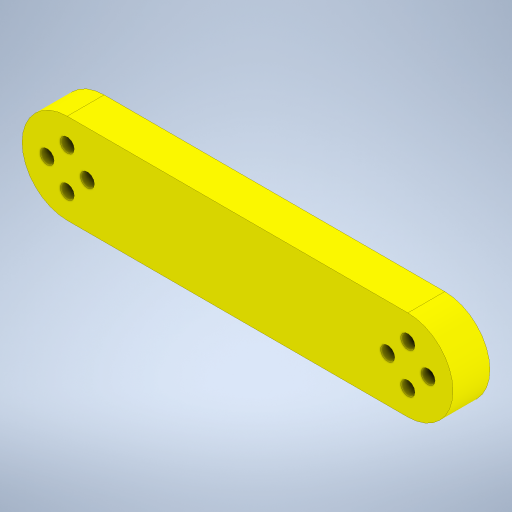
# Autodesk Inventor part: Ramie2
Saved by Autodesk Inventor 2024.2 (Build 282272000, 272)
## iProperties
Created: 2023-11-11
Part Number: Ramie2
Material: Ogólny
Document SubType Name: Modeling
Designer: nosal
Density: 1 g/cm^3
Appearance: Domyślna
Author: nosal
## iProperties of the stored document Ramie2_Drukowanie 3D.ipt
Created: 2023-11-12
Part Number: Ramie2_Drukowanie 3D
Material: Ogólny
Document SubType Name: Modeling
Designer: nosal
Density: 1 g/cm^3
Appearance: Domyślna
Author: nosal
Autodesk Inventor part; units mm, degrees
ref_plane "YZ Plane" through (0, 0, 0) normal (1, 0, 0) x (0, 1, 0)
ref_plane "XZ Plane" through (0, 0, 0) normal (0, 1, 0) x (-1, 0, 0)
sketch "Szkic1" plane through (0, 0, 0) normal (0, 0, 1) x (1, 0, 0)
  circle A0 centre (0, 0) radius 3.5
  circle A1 centre (0, 0) radius 15.9
  circle A2 centre (0, 0) radius 11.5
  line L0 (0, -15.9) -> (-60, -15.9)
  line L1 (0, 15.9) -> (-60, 15.9)
  line L2 (-60, 15.9) -> (-60, -15.9)
  point P0 (0, 7.1)
  point P1 (-7.1, 0)
  point P2 (7.1, 0)
  point P3 (0, -7.1)
  dimension "d0" = 7
  dimension "d1" = 7.1
  dimension "d2" = 7.1
  dimension "d3" = 7.1
  dimension "d4" = 7.1
  dimension "d5" = 31.8
  dimension "d6" = 23
  dimension "d23" = 60
  constraints: 6 end point, 3 centre point, 3 coincident, 2 horizontal, 2 point on circle, 1 perpendicular, 1 tangent
  measures "d0" diameter of A0
  measures "d1" distance of point (0, 0) point (0, 7.1)
  measures "d2" distance of point (7.1, 0) point (0, 0)
  measures "d3" distance of point (0, -7.1) point (0, 0)
  measures "d4" distance of point (-7.1, 0) point (0, 0)
  measures "d5" diameter of A1
  measures "d6" diameter of A2
  measures "d23" distance of L0.start L0.end
extrude "Wyciągnięcie proste1" add sketch "Szkic1" along normal blind 10 contours A0 | A1 | A1 L0 L2 L1 | A2
extrude "Wyciągnięcie proste2" cut sketch "Szkic1" along normal blind 2 contours A2
extrude "Wyciągnięcie proste3" cut sketch "Szkic1" along normal blind 3 contours A0
hole "Otwór1" at (0, 7.1, 0) at (-7.1, 0, 0) at (7.1, 0, 0) at (0, -7.1, 0) direction (0, 0, 1) diameter 1.567 end through all thread size "M2x0.4" designation "M2" class "6H" standard "GB Metric profile"
sketch "Szkic2" plane through (0, 0, 0) normal (0, 0, -1) x (0, -1, 0)
  arc A0 (-15.9, 0) -> (15.9, 0) centre (0, 0) ccw projected
  circle A1 centre (0, 0) radius 11.5 projected
  circle A2 centre (0, 0) radius 13.9
  line L0 (15.9, 60) -> (15.9, 0) projected
  line L1 (-15.9, 60) -> (15.9, 60) projected
  line L2 (-15.9, 0) -> (-15.9, 60) projected
  dimension "d20" = 2
  constraints: 1 centre point
  measures "d20" radial gap between concentric circles of A0 A2
extrude "Wyciągnięcie proste4" add sketch "Szkic2" along normal blind 3 contours L2 L1 L0 A0
ref_plane "Płaszczyzna konstrukcyjna2" through (-60, 15.9, 10) normal (1, 0, 0) x (0, -1, 0)
mirror "Odbij1" about plane through (-60, 15.9, 0) normal (-1, 0, 0) of "Wyciągnięcie proste4", "Otwór1", "Wyciągnięcie proste1", "Wyciągnięcie proste2"
sketch "Szkic4" plane through (-120, 0, 0) normal (0, 0, -1) x (-1, 0, 0)
  circle A0 centre (0, 0) radius 3.5 projected
  point P0 (-120, 0)
extrude "Wyciągnięcie proste5" cut sketch "Szkic4" against normal blind 3
sketch "Szkic5" plane through (0, 0, 10) normal (0, 0, 1) x (1, 0, 0)
  circle A0 centre (-127.1, 0) radius 0.7835 projected
  circle A1 centre (-120, -7.1) radius 0.7835 projected
  circle A2 centre (-112.9, 0) radius 0.7835 projected
  circle A3 centre (-120, 7.1) radius 0.7835 projected
  circle A4 centre (7.1, 0) radius 0.7835 projected
  circle A5 centre (0, 7.1) radius 0.7835 projected
  circle A6 centre (-7.1, 0) radius 0.7835 projected
  circle A7 centre (0, -7.1) radius 0.7835 projected
  arc A8 (0, -15.9) -> (0, 15.9) centre (0, 0) ccw projected
  line L0 (0, 15.9) -> (-120, 15.9) projected
  arc A9 (-120, 15.9) -> (-120, -15.9) centre (-120, 0) ccw projected
  line L1 (0, -15.9) -> (-120, -15.9) projected
  circle A10 centre (0, 7.1) radius 2.5
  circle A11 centre (7.1, 0) radius 2.5
  circle A12 centre (0, -7.1) radius 2.5
  circle A13 centre (-7.1, 0) radius 2.5
  circle A14 centre (-120, 7.1) radius 2.5
  circle A15 centre (-112.9, 0) radius 2.5
  circle A16 centre (-120, -7.1) radius 2.5
  circle A17 centre (-127.1, 0) radius 2.5
  dimension "d27" = 5
  dimension "d28" = 5
  dimension "d29" = 5
  dimension "d30" = 5
  dimension "d31" = 5
  dimension "d32" = 5
  dimension "d33" = 5
  dimension "d34" = 5
  constraints: 8 centre point, 8 coincident
  measures "d27" diameter of A10
  measures "d28" diameter of A11
  measures "d29" diameter of A12
  measures "d30" diameter of A13
  measures "d31" diameter of A14
  measures "d32" diameter of A15
  measures "d33" diameter of A16
  measures "d34" diameter of A17
extrude "Wyciągnięcie proste6" cut sketch "Szkic5" against normal blind 6 contours A0 | A1 | A2 | A3 | A4 | A5 | A6 | A7 | A10 | A11 | A12 | A13 | A14 | A15 | A16 | A17
equation "\"d2\" = d1"
equation "\"d3\" = d2"
equation "\"d4\" = d1"
equation "\"d18\" = d1"
